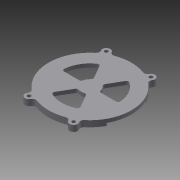
# Autodesk Inventor part: bottom_shield
Saved by Autodesk Inventor 2014 SP2 (Build 180246200, 246)
## iProperties
Created: 2015-11-29
Part Number: bottom_shield
Material: Generic
Document SubType Name: Modeling
Designer: schrluka
Density: 1 g/cm^3
Appearance: Default
Author: schrluka
Autodesk Inventor part; units mm, degrees
ref_plane "YZ Plane" through (0, 0, 0) normal (1, 0, 0) x (0, 1, 0)
ref_plane "XZ Plane" through (0, 0, 0) normal (0, 1, 0) x (-1, 0, 0)
ref_plane "XY Plane" through (0, 0, 0) normal (0, 0, 1) x (1, 0, 0)
sketch "Sketch1" plane through (0, 0, 0) normal (0, 0, 1) x (1, 0, 0)
  circle A0 centre (31.0235, 53.7343) radius 2.5 projected
  arc A1 (33.3294, 58.6976) -> (26.329, 56.4627) centre (30.8605, 54.3496) ccw projected
  arc A2 (20.0536, 53.8897) -> (26.329, 56.4627) centre (21.7974, 58.5758) ccw projected
  arc A3 (20.0536, 53.8897) -> (-20.0536, 53.8897) centre (0, 0) ccw projected
  arc A4 (-26.329, 56.4627) -> (-20.0536, 53.8897) centre (-21.7974, 58.5758) ccw projected
  arc A5 (-26.329, 56.4627) -> (-33.3294, 58.6976) centre (-30.8605, 54.3496) ccw projected
  arc A6 (-33.3294, 58.6976) -> (-34.1689, 58.2129) centre (0, 0) ccw projected
  arc A7 (-34.1689, 58.2129) -> (-35.7336, 51.0329) centre (-31.6379, 53.9008) ccw projected
  arc A8 (-36.643, 44.3118) -> (-35.7336, 51.0329) centre (-39.8294, 48.165) ccw projected
  arc A9 (-36.643, 44.3118) -> (-50.486, 27.5211) centre (0, 0) ccw projected
  line L0 (-50.486, 27.5211) -> (-42.3419, 27.5211) projected
  arc A10 (42.3419, 27.5211) -> (-42.3419, 27.5211) centre (0, 0) ccw projected
  line L1 (42.3419, 27.5211) -> (50.486, 27.5211) projected
  arc A11 (50.486, 27.5211) -> (36.643, 44.3118) centre (0, 0) ccw projected
  arc A12 (35.7336, 51.0329) -> (36.643, 44.3118) centre (39.8294, 48.165) ccw projected
  arc A13 (35.7336, 51.0329) -> (34.1689, 58.2129) centre (31.6379, 53.9008) ccw projected
  arc A14 (34.1689, 58.2129) -> (33.3294, 58.6976) centre (0, 0) ccw projected
  circle A15 centre (-31.0235, 53.7343) radius 2.5 projected
  arc A16 (26.329, -56.4627) -> (33.3294, -58.6976) centre (30.8605, -54.3496) ccw projected
  arc A17 (33.3294, -58.6976) -> (34.1689, -58.2129) centre (0, 0) ccw projected
  arc A18 (34.1689, -58.2129) -> (35.7336, -51.0329) centre (31.6379, -53.9008) ccw projected
  arc A19 (36.643, -44.3118) -> (35.7336, -51.0329) centre (39.8294, -48.165) ccw projected
  arc A20 (36.643, -44.3118) -> (50.486, -27.5211) centre (0, 0) ccw projected
  line L2 (50.486, -27.5211) -> (42.3419, -27.5211) projected
  arc A21 (-42.3419, -27.5211) -> (42.3419, -27.5211) centre (0, 0) ccw projected
  line L3 (-42.3419, -27.5211) -> (-50.486, -27.5211) projected
  arc A22 (-50.486, -27.5211) -> (-36.643, -44.3118) centre (0, 0) ccw projected
  arc A23 (-35.7336, -51.0329) -> (-36.643, -44.3118) centre (-39.8294, -48.165) ccw projected
  arc A24 (-35.7336, -51.0329) -> (-34.1689, -58.2129) centre (-31.6379, -53.9008) ccw projected
  arc A25 (-34.1689, -58.2129) -> (-33.3294, -58.6976) centre (0, 0) ccw projected
  arc A26 (-33.3294, -58.6976) -> (-26.329, -56.4627) centre (-30.8605, -54.3496) ccw projected
  arc A27 (-20.0536, -53.8897) -> (-26.329, -56.4627) centre (-21.7974, -58.5758) ccw projected
  arc A28 (-20.0536, -53.8897) -> (20.0536, -53.8897) centre (0, 0) ccw projected
  arc A29 (26.329, -56.4627) -> (20.0536, -53.8897) centre (21.7974, -58.5758) ccw projected
  circle A30 centre (31.0235, -53.7343) radius 2.5 projected
  circle A31 centre (-31.0235, -53.7343) radius 2.5 projected
extrude "Extrusion1" add sketch "Sketch1" along normal blind 3.5
sketch "Sketch2" plane through (0, 0, 3.5) normal (0, 0, 1) x (1, 0, 0)
  circle A0 centre (-31.0235, 53.7343) radius 2.5 projected
  circle A1 centre (31.0235, 53.7343) radius 2.5 projected
  arc A2 (33.3294, 58.6976) -> (26.329, 56.4627) centre (30.8605, 54.3496) ccw projected
  arc A3 (20.0536, 53.8897) -> (26.329, 56.4627) centre (21.7974, 58.5758) ccw projected
  arc A4 (20.0536, 53.8897) -> (-20.0536, 53.8897) centre (0, 0) ccw projected
  arc A5 (-26.329, 56.4627) -> (-20.0536, 53.8897) centre (-21.7974, 58.5758) ccw projected
  arc A6 (-26.329, 56.4627) -> (-33.3294, 58.6976) centre (-30.8605, 54.3496) ccw projected
  arc A7 (-33.3294, 58.6976) -> (-34.1689, 58.2129) centre (0, 0) ccw projected
  arc A8 (-34.1689, 58.2129) -> (-35.7336, 51.0329) centre (-31.6379, 53.9008) ccw projected
  arc A9 (-36.643, 44.3118) -> (-35.7336, 51.0329) centre (-39.8294, 48.165) ccw projected
  arc A10 (-36.643, 44.3118) -> (-50.486, 27.5211) centre (0, 0) ccw projected
  line L0 (-50.486, 27.5211) -> (-42.3419, 27.5211) projected
  arc A11 (42.3419, 27.5211) -> (-42.3419, 27.5211) centre (0, 0) ccw projected
  line L1 (42.3419, 27.5211) -> (50.486, 27.5211) projected
  arc A12 (50.486, 27.5211) -> (36.643, 44.3118) centre (0, 0) ccw projected
  arc A13 (35.7336, 51.0329) -> (36.643, 44.3118) centre (39.8294, 48.165) ccw projected
  arc A14 (35.7336, 51.0329) -> (34.1689, 58.2129) centre (31.6379, 53.9008) ccw projected
  arc A15 (34.1689, 58.2129) -> (33.3294, 58.6976) centre (0, 0) ccw projected
  circle A16 centre (-31.0235, -53.7343) radius 2.5 projected
  circle A17 centre (31.0235, -53.7343) radius 2.5 projected
  arc A18 (26.329, -56.4627) -> (33.3294, -58.6976) centre (30.8605, -54.3496) ccw projected
  arc A19 (33.3294, -58.6976) -> (34.1689, -58.2129) centre (0, 0) ccw projected
  arc A20 (34.1689, -58.2129) -> (35.7336, -51.0329) centre (31.6379, -53.9008) ccw projected
  arc A21 (36.643, -44.3118) -> (35.7336, -51.0329) centre (39.8294, -48.165) ccw projected
  arc A22 (36.643, -44.3118) -> (50.486, -27.5211) centre (0, 0) ccw projected
  line L2 (50.486, -27.5211) -> (42.3419, -27.5211) projected
  arc A23 (-42.3419, -27.5211) -> (42.3419, -27.5211) centre (0, 0) ccw projected
  line L3 (-42.3419, -27.5211) -> (-50.486, -27.5211) projected
  arc A24 (-50.486, -27.5211) -> (-36.643, -44.3118) centre (0, 0) ccw projected
  arc A25 (-35.7336, -51.0329) -> (-36.643, -44.3118) centre (-39.8294, -48.165) ccw projected
  arc A26 (-35.7336, -51.0329) -> (-34.1689, -58.2129) centre (-31.6379, -53.9008) ccw projected
  arc A27 (-34.1689, -58.2129) -> (-33.3294, -58.6976) centre (0, 0) ccw projected
  arc A28 (-33.3294, -58.6976) -> (-26.329, -56.4627) centre (-30.8605, -54.3496) ccw projected
  arc A29 (-20.0536, -53.8897) -> (-26.329, -56.4627) centre (-21.7974, -58.5758) ccw projected
  arc A30 (-20.0536, -53.8897) -> (20.0536, -53.8897) centre (0, 0) ccw projected
  arc A31 (26.329, -56.4627) -> (20.0536, -53.8897) centre (21.7974, -58.5758) ccw projected
  arc A32 (-50.486, 27.5211) -> (-50.486, -27.5211) centre (0, 0) ccw
  arc A33 (50.486, -27.5211) -> (50.486, 27.5211) centre (0, 0) ccw
  line L4 (-18.0807, 31.3168) -> (-7.6035, 13.1696) projected
  arc A34 (-22.3885, 32.2819) -> (-39.1512, 3.248) centre (0, 0) ccw projected
  line L5 (-15.2069, 0) -> (-36.1615, 0) projected
  line L6 (-18.0807, -31.3168) -> (-7.6035, -13.1696) projected
  line L7 (7.6035, -13.1696) -> (18.0807, -31.3168) projected
  arc A35 (-16.7627, -35.53) -> (16.7627, -35.53) centre (0, 0) ccw projected
  line L8 (36.1615, 0) -> (15.2069, 0) projected
  line L9 (7.6035, 13.1696) -> (18.0807, 31.3168) projected
  arc A36 (39.1512, 3.248) -> (22.3885, 32.2819) centre (0, 0) ccw projected
  arc A37 (12.2636, 2.4194) -> (8.227, 9.4109) centre (0, 0) ccw projected
  arc A38 (-8.227, 9.4109) -> (-12.2636, 2.4194) centre (0, 0) ccw projected
  arc A39 (-4.0366, -11.8303) -> (4.0366, -11.8303) centre (0, 0) ccw projected
  arc A40 (-18.0807, 31.3168) -> (-22.3885, 32.2819) centre (-20.6788, 29.8168) ccw projected
  arc A41 (-39.1512, 3.248) -> (-36.1615, 0) centre (-36.1615, 3) ccw projected
  arc A42 (-15.2069, 0) -> (-12.2636, 2.4194) centre (-15.2069, 3) ccw projected
  arc A43 (-8.227, 9.4109) -> (-7.6035, 13.1696) centre (-10.2015, 11.6696) ccw projected
  spline S0 degree 3 poles (8.227, 9.4109) (8.2253, 9.4125) (8.2235, 9.414) (7.9828, 9.6254) (7.7777, 9.8729) (7.4513, 10.4284) (7.3317, 10.735) (7.19, 11.4166) (7.1804, 11.7904) (7.3007, 12.5134) (7.4219, 12.855) (7.6035, 13.1696) knots -0.433605 -0.433605 -0.433605 -0.433605 -0.432845 -0.432845 -0.329157 -0.329157 -0.224657 -0.224657 -0.109223 -0.109223 0 0 0 0 projected
  arc A44 (22.3885, 32.2819) -> (18.0807, 31.3168) centre (20.6788, 29.8168) ccw projected
  arc A45 (36.1615, 0) -> (39.1512, 3.248) centre (36.1615, 3) ccw projected
  arc A46 (12.2636, 2.4194) -> (15.2069, 0) centre (15.2069, 3) ccw projected
  arc A47 (7.6035, -13.1696) -> (4.0366, -11.8303) centre (5.0054, -14.6696) ccw projected
  arc A48 (-4.0366, -11.8303) -> (-7.6035, -13.1696) centre (-5.0054, -14.6696) ccw projected
  arc A49 (-18.0807, -31.3168) -> (-16.7627, -35.53) centre (-15.4827, -32.8168) ccw projected
  arc A50 (16.7627, -35.53) -> (18.0807, -31.3168) centre (15.4827, -32.8168) ccw projected
  circle A51 centre (0, 0) radius 4.5 projected
  constraints: 4 point on circle, 2 centre point, 2 coincident
extrude "Extrusion2" add sketch "Sketch2" along normal blind 5
body "Solid1"
